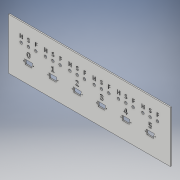
# Autodesk Inventor part: front
Saved by Autodesk Inventor 2017 (Build 210142000, 142)
## iProperties
Created: 2016-09-19
Part Number: front
Material: Generic
Document SubType Name: Modeling
Designer: Darien Morrow
Density: 1 g/cm^3
Appearance: Default
Author: Darien Morrow
Autodesk Inventor part; units mm, degrees
(part 1 of 2)
ref_plane "YZ Plane" through (0, 0, 0) normal (1, 0, 0) x (0, 1, 0)
ref_plane "XZ Plane" through (0, 0, 0) normal (0, 1, 0) x (-1, 0, 0)
ref_plane "XY Plane" through (0, 0, 0) normal (0, 0, 1) x (1, 0, 0)
sketch "Sketch1" plane through (0, 0, 0) normal (0, 0, 1) x (1, 0, 0)
  line L0 (-211.1375, -66.675) -> (211.1375, -66.675)
  line L1 (211.1375, -66.675) -> (211.1375, 66.675)
  line L2 (211.1375, 66.675) -> (-211.1375, 66.675)
  line L3 (-211.1375, 66.675) -> (-211.1375, -66.675)
  line L4 (-211.1375, -66.675) -> (211.1375, 66.675) construction
  line L5 (211.1375, -66.675) -> (-211.1375, 66.675) construction
  point P0 (0, 0)
  dimension "d0" = 133.35
  dimension "d1" = 422.275
  constraints: 12 end point, 2 midpoint, 2 parallel, 1 horizontal, 1 perpendicular
  measures "d0" distance between parallel lines of L0 L2
  measures "d1" distance between parallel lines of L1 L3
extrude "Extrusion1" add sketch "Sketch1" along normal blind 3.175
sketch "Sketch2" plane through (0, 0, 3.175) normal (0, 0, 1) x (1, 0, 0)
  line L0 (211.1375, -66.675) -> (211.1375, 66.675) projected
  line L1 (-211.1375, 19.05) -> (211.1375, 19.05)
  line L2 (211.1375, 19.05) -> (211.1375, -19.05)
  line L3 (211.1375, -19.05) -> (-211.1375, -19.05)
  line L4 (-211.1375, -19.05) -> (-211.1375, 19.05)
  line L5 (-211.1375, 19.05) -> (211.1375, -19.05) construction
  line L6 (211.1375, 19.05) -> (-211.1375, -19.05) construction
  point P0 (0, 0)
  point P1 (19.05, -19.05)
  point P2 (44.45, -19.05)
  point P3 (82.55, -19.05)
  point P4 (107.95, -19.05)
  point P5 (146.05, -19.05)
  point P6 (171.45, -19.05)
  point P7 (-19.05, -19.05)
  point P8 (-44.45, -19.05)
  point P9 (-82.55, -19.05)
  point P10 (-107.95, -19.05)
  point P11 (-146.05, -19.05)
  point P12 (-171.45, -19.05)
  dimension "d4" = 19.05
  dimension "d6" = 25.4
  dimension "d7" = 38.1
  dimension "d8" = 25.4
  dimension "d9" = 38.1
  dimension "d10" = 25.4
  dimension "d12" = 25.4
  dimension "d13" = 38.1
  dimension "d14" = 25.4
  dimension "d15" = 38.1
  dimension "d16" = 25.4
  constraints: 10 end point, 2 horizontal, 2 midpoint, 1 parallel, 1 perpendicular, 1 point on line, 15 other
  measures "d6" distance of point (44.45, -19.05) point (19.05, -19.05)
  measures "d7" distance of point (82.55, -19.05) point (44.45, -19.05)
  measures "d8" distance of point (107.95, -19.05) point (82.55, -19.05)
  measures "d9" distance of point (146.05, -19.05) point (107.95, -19.05)
  measures "d10" distance of point (171.45, -19.05) point (146.05, -19.05)
  measures "d12" distance of point (-44.45, -19.05) point (-19.05, -19.05)
  measures "d13" distance of point (-82.55, -19.05) point (-44.45, -19.05)
  measures "d14" distance of point (-107.95, -19.05) point (-82.55, -19.05)
  measures "d15" distance of point (-146.05, -19.05) point (-107.95, -19.05)
  measures "d16" distance of point (-171.45, -19.05) point (-146.05, -19.05)
hole "Hole1" at (19.05, -19.05, 3.175) at (44.45, -19.05, 3.175) at (82.55, -19.05, 3.175) at (107.95, -19.05, 3.175) at (146.05, -19.05, 3.175) at (171.45, -19.05, 3.175) at (-19.05, -19.05, 3.175) at (-44.45, -19.05, 3.175) at (-82.55, -19.05, 3.175) at (-107.95, -19.05, 3.175) at (-146.05, -19.05, 3.175) at (-171.45, -19.05, 3.175) direction (0, 0, -1) diameter 2.159 end through all
sketch "Sketch3" plane through (0, 0, 3.175) normal (0, 0, 1) x (1, 0, 0)
  circle A0 centre (-146.05, -19.05) radius 1.0795 projected
  line L0 (-211.1375, -66.675) -> (211.1375, -66.675) projected
  line L1 (-167.4813, -25.0031) -> (-150.0188, -25.0031)
  line L2 (-150.0188, -13.0969) -> (-167.4813, -13.0969)
  line L3 (-167.4813, -25.0031) -> (-150.0188, -13.0969) construction
  line L4 (-150.0188, -25.0031) -> (-167.4813, -13.0969) construction
  line L5 (-150.0188, -25.0031) -> (-148.4313, -13.0969)
  line L6 (-167.4813, -25.0031) -> (-169.0688, -13.0969)
  line L7 (-169.0688, -13.0969) -> (-167.4813, -13.0969)
  line L8 (-150.0188, -13.0969) -> (-148.4313, -13.0969)
  line L9 (-161.2761, -3.996) -> (-100.8121, -3.996)
  line L10 (-86.5188, -13.0969) -> (-103.9813, -13.0969)
  line L11 (-105.5688, -13.0969) -> (-103.9813, -13.0969)
  line L12 (-103.9813, -25.0031) -> (-105.5688, -13.0969)
  line L13 (-103.9813, -25.0031) -> (-86.5188, -25.0031)
  line L14 (-86.5188, -25.0031) -> (-84.9313, -13.0969)
  line L15 (-86.5188, -13.0969) -> (-84.9313, -13.0969)
  line L16 (-23.0188, -13.0969) -> (-40.4813, -13.0969)
  line L17 (-42.0688, -13.0969) -> (-40.4813, -13.0969)
  line L18 (-40.4813, -25.0031) -> (-42.0688, -13.0969)
  line L19 (-40.4813, -25.0031) -> (-23.0188, -25.0031)
  line L20 (-23.0188, -25.0031) -> (-21.4313, -13.0969)
  line L21 (-23.0188, -13.0969) -> (-21.4313, -13.0969)
  line L22 (40.4812, -13.0969) -> (23.0187, -13.0969)
  line L23 (21.4312, -13.0969) -> (23.0187, -13.0969)
  line L24 (23.0187, -25.0031) -> (21.4312, -13.0969)
  line L25 (23.0187, -25.0031) -> (40.4812, -25.0031)
  line L26 (40.4812, -25.0031) -> (42.0687, -13.0969)
  line L27 (40.4812, -13.0969) -> (42.0687, -13.0969)
  line L28 (103.9812, -13.0969) -> (86.5187, -13.0969)
  line L29 (84.9312, -13.0969) -> (86.5187, -13.0969)
  line L30 (86.5187, -25.0031) -> (84.9312, -13.0969)
  line L31 (86.5187, -25.0031) -> (103.9812, -25.0031)
  line L32 (103.9812, -25.0031) -> (105.5687, -13.0969)
  line L33 (103.9812, -13.0969) -> (105.5687, -13.0969)
  line L34 (167.4813, -13.0969) -> (150.0187, -13.0969)
  line L35 (148.4312, -13.0969) -> (150.0187, -13.0969)
  line L36 (150.0187, -25.0031) -> (148.4312, -13.0969)
  line L37 (150.0187, -25.0031) -> (167.4813, -25.0031)
  line L38 (167.4813, -25.0031) -> (169.0687, -13.0969)
  line L39 (167.4813, -13.0969) -> (169.0687, -13.0969)
  point P0 (0, 0)
  point P1 (-158.75, -19.05)
  dimension "d24" = 12.7
  dimension "d25" = 47.625
  dimension "d26" = 17.4625
  dimension "d27" = 11.9062
  dimension "d28" = 1.5875
  dimension "d29" = 1.5875
  dimension "d32" = 63.5
  constraints: 78 end point, 4 horizontal, 2 equal length, 2 midpoint, 60 other
  measures "d24" distance of point (-158.75, -19.05) A0.centre
  measures "d25" distance from line of point (-158.75, -19.05) L0
  measures "d26" distance of L2.end L2.start
  measures "d27" distance between parallel lines of L1 L2
  measures "d28" distance of L5.end L2.start
  measures "d29" distance of L2.end L6.end
  measures "d32" distance of L2.start L10.start
extrude "Extrusion2" cut sketch "Sketch3" against normal blind 25.4 contours L6 L7 L2 L8 L5 L1 | L15 L14 L13 L12 L11 L10 | L21 L20 L19 L18 L17 L16 | L27 L26 L25 L24 L23 L22 | L33 L32 L31 L30 L29 L28 | L39 L38 L37 L36 L35 L34
sketch "Sketch4" plane through (0, 0, 3.175) normal (0, 0, 1) x (1, 0, 0)
  line L0 (211.1375, 66.675) -> (-211.1375, 66.675) projected
  line L1 (177.8, -19.05) -> (-177.8, -19.05)
  line L2 (-177.8, -19.05) -> (-177.8, 19.05)
  line L3 (-177.8, 19.05) -> (177.8, 19.05)
  line L4 (177.8, 19.05) -> (177.8, -19.05)
  line L5 (177.8, -19.05) -> (-177.8, 19.05) construction
  line L6 (-177.8, -19.05) -> (177.8, 19.05) construction
  point P0 (0, 0)
  point P1 (-158.75, 19.05)
  point P2 (-139.7, 19.05)
  point P3 (-114.3, 19.05)
  point P4 (-95.25, 19.05)
  point P5 (-76.2, 19.05)
  point P6 (-50.8, 19.05)
  point P7 (-31.75, 19.05)
  point P8 (-12.7, 19.05)
  point P9 (12.7, 19.05)
  point P10 (31.75, 19.05)
  point P11 (50.8, 19.05)
  point P12 (76.2, 19.05)
  point P13 (95.25, 19.05)
  point P14 (114.3, 19.05)
  point P15 (139.7, 19.05)
  point P16 (158.75, 19.05)
  point P17 (177.8, 19.05)
  dimension "d40" = 38.1
  dimension "d41" = 355.6
  dimension "d42" = 19.05
  dimension "d43" = 19.05
  dimension "d46" = 63.5
  constraints: 12 end point, 2 horizontal, 2 midpoint, 2 parallel, 2 point on line, 1 coincident, 1 perpendicular, 15 other
  measures "d40" distance between parallel lines of L1 L3
  measures "d41" distance between parallel lines of L4 L2
  measures "d42" distance of point (-158.75, 19.05) L2.end
  measures "d43" distance of point (-139.7, 19.05) point (-158.75, 19.05)
  measures "d46" distance of L2.end point (-114.3, 19.05)
hole "Hole2" at (-177.8, 19.05, 3.175) at (-158.75, 19.05, 3.175) at (-139.7, 19.05, 3.175) at (-95.25, 19.05, 3.175) at (-76.2, 19.05, 3.175) at (-31.75, 19.05, 3.175) at (-12.7, 19.05, 3.175) at (31.75, 19.05, 3.175) at (50.8, 19.05, 3.175) at (95.25, 19.05, 3.175) at (114.3, 19.05, 3.175) at (158.75, 19.05, 3.175) at (177.8, 19.05, 3.175) at (-50.8, 19.05, 3.175) at (-114.3, 19.05, 3.175) at (12.7, 19.05, 3.175) at (76.2, 19.05, 3.175) at (139.7, 19.05, 3.175) direction (0, 0, -1) diameter 7 end through all
sketch "Sketch5" plane through (0, 0, 3.175) normal (0, 0, 1) x (1, 0, 0)
  line L0 (-163.6339, 6.5797) -> (-140.462, 6.5797) construction
  line L1 (-140.462, 6.5797) -> (-140.462, -4.8632) construction
  line L2 (-140.462, -4.8632) -> (-163.6339, -4.8632) construction
  line L3 (-163.6339, -4.8632) -> (-163.6339, 6.5797) construction
  line L4 (-100.7374, 6.1393) -> (-89.5805, 6.1393) construction
  line L5 (-89.5805, 6.1393) -> (-89.5805, -9.0226) construction
  line L6 (-89.5805, -9.0226) -> (-100.7374, -9.0226) construction
  line L7 (-100.7374, -9.0226) -> (-100.7374, 6.1393) construction
  circle A0 centre (158.75, 19.05) radius 3.5 projected
  line L8 (-211.1375, 66.675) -> (-211.1375, -66.675) projected
  line L9 (-36.8587, 6.6086) -> (-14.4346, 6.6086) construction
  line L10 (-14.4346, 6.6086) -> (-14.4346, -5.5869) construction
  line L11 (-14.4346, -5.5869) -> (-36.8587, -5.5869) construction
  line L12 (-36.8587, -5.5869) -> (-36.8587, 6.6086) construction
  line L13 (27.033, 6.6307) -> (37.1692, 6.6307) construction
  line L14 (37.1692, 6.6307) -> (37.1692, -6.4628) construction
  line L15 (37.1692, -6.4628) -> (27.033, -6.4628) construction
  line L16 (27.033, -6.4628) -> (27.033, 6.6307) construction
  line L17 (89.8174, 6.414) -> (98.2756, 6.414) construction
  line L18 (98.2756, 6.414) -> (98.2756, 0.1196) construction
  line L19 (98.2756, 0.1196) -> (89.8174, 0.1196) construction
  line L20 (89.8174, 0.1196) -> (89.8174, 6.414) construction
  line L21 (153.7586, 6.5556) -> (163.8948, 6.5556) construction
  line L22 (163.8948, 6.5556) -> (163.8948, -6.3113) construction
  line L23 (163.8948, -6.3113) -> (153.7586, -6.3113) construction
  line L24 (153.7586, -6.3113) -> (153.7586, 6.5556) construction
  spline S0 degree 2 poles (-154.0344, 0.0806) (-154.0344, -1.4338) (-154.5233, -3.8784) (-155.6323, -5.5956) (-157.3972, -6.5138) (-158.6731, -6.5138) knots 0 0 0 1 2 3 4 4 4
  spline S1 degree 2 poles (-158.6731, -6.5138) (-159.973, -6.5138) (-161.6782, -5.6195) (-162.668, -3.95) (-163.0734, -1.5412) (-163.0734, -0.0148) knots 0 0 0 1 2 3 4 4 4
  spline S2 degree 2 poles (-163.0734, -0.0148) (-163.0734, 1.4878) (-162.5726, 3.9443) (-161.4755, 5.6615) (-159.6987, 6.5797) (-158.4346, 6.5797) knots 0 0 0 1 2 3 4 4 4
  spline S3 degree 2 poles (-158.4346, 6.5797) (-157.1348, 6.5797) (-155.4177, 5.6853) (-154.4279, 4.0158) (-154.0344, 1.607) (-154.0344, 0.0806) knots 0 0 0 1 2 3 4 4 4
  spline S4 degree 2 poles (-156.6221, -0.0386) (-156.6221, 0.8557) (-156.7175, 2.239) (-156.9202, 3.2526) (-157.2302, 3.9562) (-157.6595, 4.3736) (-158.2081, 4.5525) (-158.542, 4.5525) knots 0 0 0 1 2 3 4 5 6 6 6
  spline S5 degree 2 poles (-158.542, 4.5525) (-159.1144, 4.5525) (-159.8656, 3.992) (-160.3069, 2.883) (-160.4857, 1.2135) (-160.4857, 0.1164) knots 0 0 0 1 2 3 4 4 4
  spline S6 degree 2 poles (-160.4857, 0.1164) (-160.4857, -1.243) (-160.2711, -3.0079) (-159.806, -4.0573) (-159.0905, -4.4747) (-158.5777, -4.4747) knots 0 0 0 1 2 3 4 4 4
  spline S7 degree 2 poles (-158.5777, -4.4747) (-158.1962, -4.4747) (-157.6118, -4.2243) (-157.1706, -3.7353) (-156.8725, -2.996) (-156.6936, -2.0182) (-156.6221, -0.7899) (-156.6221, -0.0386) knots 0 0 0 1 2 3 4 5 6 6 6
  spline S8 degree 2 poles (-91.5075, -5.6186) (-91.5075, -5.8929) (-91.5672, -6.2745) (-91.6745, -6.5011) (-91.8057, -6.5965) (-91.9011, -6.5965) knots 0 0 0 1 2 3 4 4 4
  line L25 (-91.9011, -6.5965) -> (-98.8771, -6.5965)
  spline S9 degree 2 poles (-98.8771, -6.5965) (-98.9606, -6.5965) (-99.0918, -6.5011) (-99.1991, -6.2745) (-99.2587, -5.8929) (-99.2587, -5.6186) knots 0 0 0 1 2 3 4 4 4
  spline S10 degree 2 poles (-99.2587, -5.6186) (-99.2587, -5.3444) (-99.211, -4.9628) (-99.1037, -4.7243) (-98.9606, -4.6169) (-98.8771, -4.6169) knots 0 0 0 1 2 3 4 4 4
  line L26 (-98.8771, -4.6169) -> (-96.5279, -4.6169)
  line L27 (-96.5279, -4.6169) -> (-96.5279, 3.6231)
  line L28 (-96.5279, 3.6231) -> (-98.5671, 2.5022)
  spline S11 degree 2 poles (-98.5671, 2.5022) (-98.7817, 2.3949) (-99.0679, 2.3472) (-99.2349, 2.5141) (-99.2945, 2.9196) (-99.2945, 3.2892) knots 0 0 0 1 2 3 4 4 4
  spline S12 degree 2 poles (-99.2945, 3.2892) (-99.2945, 3.5277) (-99.2706, 3.8259) (-99.1991, 4.0405) (-99.056, 4.1836) (-98.9367, 4.2552) knots 0 0 0 1 2 3 4 4 4
  line L29 (-98.9367, 4.2552) -> (-96.2298, 6.0081)
  spline S13 degree 2 poles (-96.2298, 6.0081) (-96.1702, 6.0558) (-96.0271, 6.1035) (-95.7886, 6.1274) (-95.407, 6.1393) (-95.1088, 6.1393) knots 0 0 0 1 2 3 4 4 4
  spline S14 degree 2 poles (-95.1088, 6.1393) (-94.7392, 6.1393) (-94.2741, 6.1154) (-94.0475, 6.0439) (-93.9641, 5.9246) (-93.9641, 5.8412) knots 0 0 0 1 2 3 4 4 4
  line L30 (-93.9641, 5.8412) -> (-93.9641, -4.6169)
  line L31 (-93.9641, -4.6169) -> (-91.9011, -4.6169)
  spline S15 degree 2 poles (-91.9011, -4.6169) (-91.8057, -4.6169) (-91.6626, -4.7243) (-91.5552, -4.9628) (-91.5075, -5.3444) (-91.5075, -5.6186) knots 0 0 0 1 2 3 4 4 4
  spline S16 degree 2 poles (-27.5215, -5.209) (-27.5215, -5.4952) (-27.5692, -5.9006) (-27.6646, -6.151) (-27.8196, -6.2584) (-27.9269, -6.2584) knots 0 0 0 1 2 3 4 4 4
  line L32 (-27.9269, -6.2584) -> (-35.1892, -6.2584)
  spline S17 degree 2 poles (-35.1892, -6.2584) (-35.4038, -6.2584) (-35.7139, -6.1749) (-35.9166, -5.9602) (-36.0001, -5.519) (-36.0001, -5.1851) knots 0 0 0 1 2 3 4 4 4
  spline S18 degree 2 poles (-36.0001, -5.1851) (-36.0001, -4.8632) (-35.9404, -4.3981) (-35.7854, -4.0403) (-35.535, -3.6945) (-35.3442, -3.4918) knots 0 0 0 1 2 3 4 4 4
  line L33 (-35.3442, -3.4918) -> (-33.1619, -1.1426)
  spline S19 degree 2 poles (-33.1619, -1.1426) (-32.5061, -0.4629) (-31.7071, 0.6581) (-31.254, 1.5882) (-31.087, 2.3633) (-31.087, 2.7211) knots 0 0 0 1 2 3 4 4 4
  spline S20 degree 2 poles (-31.087, 2.7211) (-31.087, 3.043) (-31.2897, 3.6154) (-31.6952, 4.0447) (-32.2914, 4.2952) (-32.7088, 4.2952) knots 0 0 0 1 2 3 4 4 4
  spline S21 degree 2 poles (-32.7088, 4.2952) (-33.2812, 4.2952) (-34.1756, 4.009) (-34.8433, 3.6393) (-35.2965, 3.3412) (-35.4157, 3.3412) knots 0 0 0 1 2 3 4 4 4
  spline S22 degree 2 poles (-35.4157, 3.3412) (-35.5111, 3.3412) (-35.6304, 3.4604) (-35.7139, 3.7347) (-35.7616, 4.1878) (-35.7616, 4.5217) knots 0 0 0 1 2 3 4 4 4
  spline S23 degree 2 poles (-35.7616, 4.5217) (-35.7616, 4.7483) (-35.7377, 5.0583) (-35.6781, 5.273) (-35.5708, 5.4399) (-35.3323, 5.6784) (-34.6764, 6.0362) (-33.7224, 6.382) (-32.5657, 6.6086) (-31.9456, 6.6086) knots 0 0 0 1 2 3 4 5 6 7 8 8 8
  spline S24 degree 2 poles (-31.9456, 6.6086) (-30.9558, 6.6086) (-29.4891, 6.1077) (-28.5112, 5.2253) (-28.0342, 3.997) (-28.0342, 3.2935) knots 0 0 0 1 2 3 4 4 4
  spline S25 degree 2 poles (-28.0342, 3.2935) (-28.0342, 2.6853) (-28.2727, 1.4928) (-29.0121, 0.1095) (-30.3596, -1.56) (-31.4686, -2.6571) knots 0 0 0 1 2 3 4 4 4
  line L34 (-31.4686, -2.6571) -> (-32.9473, -4.1715)
  line L35 (-32.9473, -4.1715) -> (-27.9627, -4.1715)
  spline S26 degree 2 poles (-27.9627, -4.1715) (-27.8673, -4.1715) (-27.7003, -4.2908) (-27.5811, -4.5293) (-27.5215, -4.9347) (-27.5215, -5.209) knots 0 0 0 1 2 3 4 4 4
  spline S27 degree 2 poles (36.3225, -2.5395) (36.3225, -3.4816) (35.5951, -4.9483) (34.3072, -5.95) (32.5065, -6.4628) (31.4452, -6.4628) knots 0 0 0 1 2 3 4 4 4
  spline S28 degree 2 poles (31.4452, -6.4628) (30.8013, -6.4628) (29.6684, -6.272) (28.7979, -6.0096) (28.2255, -5.7115) (28.0586, -5.5565) (27.9632, -5.3538) (27.8916, -5.0914) (27.8678, -4.6979) (27.8678, -4.4117) knots 0 0 0 1 2 3 4 5 6 7 8 8 8
  spline S29 degree 2 poles (27.8678, -4.4117) (27.8678, -3.9347) (28.0228, -3.577) (28.1778, -3.577) knots 0 0 0 1 2 2 2
  spline S30 degree 2 poles (28.1778, -3.577) (28.2732, -3.577) (28.7621, -3.8393) (29.5015, -4.1494) (30.5032, -4.4117) (31.1352, -4.4117) knots 0 0 0 1 2 3 4 4 4
  spline S31 degree 2 poles (31.1352, -4.4117) (31.6718, -4.4117) (32.4946, -4.1613) (33.067, -3.6962) (33.3532, -3.0404) (33.3532, -2.6468) knots 0 0 0 1 2 3 4 4 4
  spline S32 degree 2 poles (33.3532, -2.6468) (33.3532, -2.2056) (33.0074, -1.502) (32.3396, -1.0012) (31.3141, -0.7269) (30.6105, -0.7269) knots 0 0 0 1 2 3 4 4 4
  line L36 (30.6105, -0.7269) -> (29.5134, -0.7269)
  spline S33 degree 2 poles (29.5134, -0.7269) (29.3942, -0.7269) (29.2153, -0.6554) (29.096, -0.4407) (29.0483, -0.0591) (29.0483, 0.239) knots 0 0 0 1 2 3 4 4 4
  spline S34 degree 2 poles (29.0483, 0.239) (29.0483, 0.5252) (29.096, 0.8829) (29.2034, 1.0737) (29.3703, 1.1572) (29.4896, 1.1572) knots 0 0 0 1 2 3 4 4 4
  line L37 (29.4896, 1.1572) -> (30.5986, 1.1572)
  spline S35 degree 2 poles (30.5986, 1.1572) (31.171, 1.1572) (32.0534, 1.4196) (32.6496, 1.9085) (32.9597, 2.6001) (32.9597, 3.0294) knots 0 0 0 1 2 3 4 4 4
  spline S36 degree 2 poles (32.9597, 3.0294) (32.9597, 3.3514) (32.745, 3.9238) (32.3277, 4.3412) (31.6599, 4.5916) (31.2067, 4.5916) knots 0 0 0 1 2 3 4 4 4
  spline S37 degree 2 poles (31.2067, 4.5916) (30.694, 4.5916) (29.7996, 4.2935) (29.0841, 3.9238) (28.5833, 3.6137) (28.464, 3.6137) knots 0 0 0 1 2 3 4 4 4
  spline S38 degree 2 poles (28.464, 3.6137) (28.3925, 3.6137) (28.2732, 3.6853) (28.1897, 3.8761) (28.154, 4.2458) (28.154, 4.5439) knots 0 0 0 1 2 3 4 4 4
  spline S39 degree 2 poles (28.154, 4.5439) (28.154, 4.7824) (28.1778, 5.1043) (28.2374, 5.319) (28.3209, 5.474) (28.5117, 5.6648) (29.1199, 6.0345) (30.0381, 6.3922) (31.2425, 6.6307) (31.9461, 6.6307) knots 0 0 0 1 2 3 4 5 6 7 8 8 8
  spline S40 degree 2 poles (31.9461, 6.6307) (32.8643, 6.6307) (34.2834, 6.2014) (35.2493, 5.3905) (35.7501, 4.21) (35.7501, 3.4587) knots 0 0 0 1 2 3 4 4 4
  spline S41 degree 2 poles (35.7501, 3.4587) (35.7501, 2.8863) (35.452, 1.8965) (34.8915, 1.1095) (34.0329, 0.561) (33.4844, 0.4298) knots 0 0 0 1 2 3 4 4 4
  line L38 (33.4844, 0.4298) -> (33.4844, 0.394)
  spline S42 degree 2 poles (33.4844, 0.394) (34.1403, 0.3225) (35.2016, -0.2022) (35.929, -0.9773) (36.3225, -1.9671) (36.3225, -2.5395) knots 0 0 0 1 2 3 4 4 4
  spline S43 degree 2 poles (99.5601, -2.6608) (99.5601, -3.1616) (99.3573, -3.6744) (99.1785, -3.6744) knots 0 0 0 1 2 2 2
  line L39 (99.1785, -3.6744) -> (98.0575, -3.6744)
  line L40 (98.0575, -3.6744) -> (98.0575, -5.9521)
  spline S44 degree 2 poles (98.0575, -5.9521) (98.0575, -6.0475) (97.9383, -6.2025) (97.6521, -6.2979) (97.1751, -6.3456) (96.8054, -6.3456) knots 0 0 0 1 2 3 4 4 4
  spline S45 degree 2 poles (96.8054, -6.3456) (96.4596, -6.3456) (95.9826, -6.2979) (95.6964, -6.2025) (95.5891, -6.0475) (95.5891, -5.9521) knots 0 0 0 1 2 3 4 4 4
  line L41 (95.5891, -5.9521) -> (95.5891, -3.6744)
  line L42 (95.5891, -3.6744) -> (90.7476, -3.6744)
  spline S46 degree 2 poles (90.7476, -3.6744) (90.6045, -3.6744) (90.3898, -3.6029) (90.2467, -3.3644) (90.1752, -2.8993) (90.1752, -2.5177) knots 0 0 0 1 2 3 4 4 4
  spline S47 degree 2 poles (90.1752, -2.5177) (90.1752, -2.2076) (90.199, -1.7545) (90.2706, -1.3729) (90.4018, -1.0509) (90.4972, -0.8601) knots 0 0 0 1 2 3 4 4 4
  line L43 (90.4972, -0.8601) -> (94.4324, 6.0682)
  spline S48 degree 2 poles (94.4324, 6.0682) (94.4801, 6.1636) (94.7186, 6.2829) (95.1359, 6.3783) (95.7799, 6.414) (96.245, 6.414) knots 0 0 0 1 2 3 4 4 4
  spline S49 degree 2 poles (96.245, 6.414) (96.7458, 6.414) (97.4374, 6.3663) (97.8667, 6.259) (98.0575, 6.104) (98.0575, 5.9967) knots 0 0 0 1 2 3 4 4 4
  line L44 (98.0575, 5.9967) -> (98.0575, -1.6233)
  line L45 (98.0575, -1.6233) -> (99.1785, -1.6233)
  spline S50 degree 2 poles (99.1785, -1.6233) (99.3335, -1.6233) (99.5601, -2.1003) (99.5601, -2.6608) knots 0 0 0 1 2 2 2
  line L46 (95.5891, 4.196) -> (95.5652, 4.196)
  line L47 (95.5652, 4.196) -> (92.2263, -1.6233)
  line L48 (92.2263, -1.6233) -> (95.5891, -1.6233)
  line L49 (95.5891, -1.6233) -> (95.5891, 4.196)
  spline S51 degree 2 poles (162.9885, -1.9826) (162.9885, -3.0081) (162.273, -4.618) (160.9732, -5.727) (159.1487, -6.3113) (158.0277, -6.3113) knots 0 0 0 1 2 3 4 4 4
  spline S52 degree 2 poles (158.0277, -6.3113) (157.4434, -6.3113) (156.394, -6.1682) (155.5473, -5.9417) (155.0107, -5.7151) (154.8438, -5.572) (154.7722, -5.3931) (154.7245, -5.1427) (154.7007, -4.773) (154.7007, -4.5226) knots 0 0 0 1 2 3 4 5 6 7 8 8 8
  spline S53 degree 2 poles (154.7007, -4.5226) (154.7007, -4.2483) (154.7365, -3.8667) (154.8319, -3.6282) (154.9392, -3.5328) (155.0227, -3.5328) knots 0 0 0 1 2 3 4 4 4
  spline S54 degree 2 poles (155.0227, -3.5328) (155.1181, -3.5328) (155.5235, -3.7594) (156.1794, -4.0337) (157.1095, -4.2603) (157.7654, -4.2603) knots 0 0 0 1 2 3 4 4 4
  spline S55 degree 2 poles (157.7654, -4.2603) (158.3378, -4.2603) (159.256, -4.0218) (159.9119, -3.509) (160.2577, -2.722) (160.2577, -2.1853) knots 0 0 0 1 2 3 4 4 4
  spline S56 degree 2 poles (160.2577, -2.1853) (160.2577, -1.7083) (159.9596, -0.9809) (159.3395, -0.4681) (158.3497, -0.2177) (157.6342, -0.2177) knots 0 0 0 1 2 3 4 4 4
  spline S57 degree 2 poles (157.6342, -0.2177) (157.0618, -0.2177) (156.1436, -0.337) (155.7262, -0.337) knots 0 0 0 1 2 2 2
  spline S58 degree 2 poles (155.7262, -0.337) (155.44, -0.337) (155.2015, -0.0508) (155.2015, 0.3308) knots 0 0 0 1 2 2 2
  line L50 (155.2015, 0.3308) -> (155.2015, 5.8282)
  spline S59 degree 2 poles (155.2015, 5.8282) (155.2015, 6.2098) (155.4996, 6.5556) (155.8335, 6.5556) knots 0 0 0 1 2 2 2
  line L51 (155.8335, 6.5556) -> (161.8198, 6.5556)
  spline S60 degree 2 poles (161.8198, 6.5556) (161.9152, 6.5556) (162.0703, 6.4364) (162.1776, 6.1859) (162.2253, 5.7686) (162.2253, 5.4704) knots 0 0 0 1 2 3 4 4 4
  spline S61 degree 2 poles (162.2253, 5.4704) (162.2253, 4.8861) (162.0226, 4.3614) (161.8198, 4.3614) knots 0 0 0 1 2 2 2
  line L52 (161.8198, 4.3614) -> (157.3361, 4.3614)
  line L53 (157.3361, 4.3614) -> (157.3361, 1.6426)
  spline S62 degree 2 poles (157.3361, 1.6426) (157.6819, 1.6783) (158.3497, 1.7022) (158.7194, 1.7022) knots 0 0 0 1 2 2 2
  spline S63 degree 2 poles (158.7194, 1.7022) (159.7449, 1.7022) (161.3428, 1.2252) (162.428, 0.295) (162.9885, -1.0763) (162.9885, -1.9826) knots 0 0 0 1 2 3 4 4 4
  point P0 (0, 0)
  constraints: 12 other
emboss "Emboss1" sketch "Sketch5" operation cut depth 1.27 direction (0, 0, -1) contours S0 S1 S2 S3 | S8 L25 S9 S10 L26 L27 L28 S11 S12 L29 S13 S14 L30 L31 S15 | S16 L32 S17 S18 L33 S19 S20 S21 S22 S23 S24 S25 L34 L35 S26 | S27 S28 S29 S30 S31 S32 L36 S33 S34 L37 S35 S36 S37 S38 S39 S40 S41 L38 S42 | S43 L39 L40 S44 S45 L41 L42 S46 S47 L43 S48 S49 L44 L45 S50 | S51 S52 S53 S54 S55 S56 S57 S58 L50 S59 L51 S60 S61 L52 L53 S62 S63
sketch "Sketch6" plane through (0, 0, 3.175) normal (0, 0, 1) x (1, 0, 0)
  line L0 (-182.5364, 38.2905) -> (-176.4863, 38.2905) construction
  line L1 (-176.4863, 38.2905) -> (-176.4863, 32.7976) construction
  line L2 (-176.4863, 32.7976) -> (-182.5364, 32.7976) construction
  line L3 (-182.5364, 32.7976) -> (-182.5364, 38.2905) construction
  line L4 (-162.3961, 38.6089) -> (-155.3038, 38.6089) construction
  line L5 (-155.3038, 38.6089) -> (-155.3038, 28.7887) construction
  line L6 (-155.3038, 28.7887) -> (-162.3961, 28.7887) construction
  line L7 (-162.3961, 28.7887) -> (-162.3961, 38.6089) construction
  line L8 (-142.813, 38.2108) -> (-135.9264, 38.2108) construction
  line L9 (-135.9264, 38.2108) -> (-135.9264, 28.6858) construction
  line L10 (-135.9264, 28.6858) -> (-142.813, 28.6858) construction
  line L11 (-142.813, 28.6858) -> (-142.813, 38.2108) construction
  line L12 (-118.6971, 38.2858) -> (-112.647, 38.2858) construction
  line L13 (-112.647, 38.2858) -> (-112.647, 32.793) construction
  line L14 (-112.647, 32.793) -> (-118.6971, 32.793) construction
  line L15 (-118.6971, 32.793) -> (-118.6971, 38.2858) construction
  line L16 (-98.5568, 38.6043) -> (-91.4644, 38.6043) construction
  line L17 (-91.4644, 38.6043) -> (-91.4644, 28.7841) construction
  line L18 (-91.4644, 28.7841) -> (-98.5568, 28.7841) construction
  line L19 (-98.5568, 28.7841) -> (-98.5568, 38.6043) construction
  line L20 (-78.9737, 38.2062) -> (-72.0871, 38.2062) construction
  line L21 (-72.0871, 38.2062) -> (-72.0871, 28.6812) construction
  line L22 (-72.0871, 28.6812) -> (-78.9737, 28.6812) construction
  line L23 (-78.9737, 28.6812) -> (-78.9737, 38.2062) construction
  line L24 (211.1375, -66.675) -> (211.1375, 66.675) projected
  circle A0 centre (12.7, 19.05) radius 3.5 projected
  line L25 (-15.5126, 28.7583) -> (-15.5126, 38.2833) construction
  line L26 (-15.5126, 38.2833) -> (-8.626, 38.2833) construction
  line L27 (-8.626, 38.2833) -> (-8.626, 28.7583) construction
  line L28 (-8.626, 28.7583) -> (-15.5126, 28.7583) construction
  line L29 (-35.0957, 28.8612) -> (-35.0957, 38.6813) construction
  line L30 (-35.0957, 38.6813) -> (-28.0033, 38.6813) construction
  line L31 (-28.0033, 38.6813) -> (-28.0033, 28.8612) construction
  line L32 (-28.0033, 28.8612) -> (-35.0957, 28.8612) construction
  line L33 (-55.236, 32.8701) -> (-55.236, 38.3629) construction
  line L34 (-55.236, 38.3629) -> (-49.1859, 38.3629) construction
  line L35 (-49.1859, 38.3629) -> (-49.1859, 32.8701) construction
  line L36 (-49.1859, 32.8701) -> (-55.236, 32.8701) construction
  line L37 (8.0094, 32.7314) -> (8.0094, 38.2242) construction
  line L38 (8.0094, 38.2242) -> (14.0594, 38.2242) construction
  line L39 (14.0594, 38.2242) -> (14.0594, 32.7314) construction
  line L40 (14.0594, 32.7314) -> (8.0094, 32.7314) construction
  line L41 (28.1497, 28.7225) -> (28.1497, 38.5426) construction
  line L42 (28.1497, 38.5426) -> (35.242, 38.5426) construction
  line L43 (35.242, 38.5426) -> (35.242, 28.7225) construction
  line L44 (35.242, 28.7225) -> (28.1497, 28.7225) construction
  line L45 (47.7327, 28.6196) -> (47.7327, 38.1446) construction
  line L46 (47.7327, 38.1446) -> (54.6193, 38.1446) construction
  line L47 (54.6193, 38.1446) -> (54.6193, 28.6196) construction
  line L48 (54.6193, 28.6196) -> (47.7327, 28.6196) construction
  line L49 (111.3017, 28.6967) -> (111.3017, 38.2217) construction
  line L50 (111.3017, 38.2217) -> (118.1883, 38.2217) construction
  line L51 (118.1883, 38.2217) -> (118.1883, 28.6967) construction
  line L52 (118.1883, 28.6967) -> (111.3017, 28.6967) construction
  line L53 (91.7186, 28.7996) -> (91.7186, 38.6197) construction
  line L54 (91.7186, 38.6197) -> (98.811, 38.6197) construction
  line L55 (98.811, 38.6197) -> (98.811, 28.7996) construction
  line L56 (98.811, 28.7996) -> (91.7186, 28.7996) construction
  line L57 (71.5783, 32.8085) -> (71.5783, 38.3013) construction
  line L58 (71.5783, 38.3013) -> (77.6284, 38.3013) construction
  line L59 (77.6284, 38.3013) -> (77.6284, 32.8085) construction
  line L60 (77.6284, 32.8085) -> (71.5783, 32.8085) construction
  line L61 (135.0934, 32.7237) -> (135.0934, 38.2165) construction
  line L62 (135.0934, 38.2165) -> (141.1434, 38.2165) construction
  line L63 (141.1434, 38.2165) -> (141.1434, 32.7237) construction
  line L64 (141.1434, 32.7237) -> (135.0934, 32.7237) construction
  line L65 (155.2337, 28.7148) -> (155.2337, 38.5349) construction
  line L66 (155.2337, 38.5349) -> (162.326, 38.5349) construction
  line L67 (162.326, 38.5349) -> (162.326, 28.7148) construction
  line L68 (162.326, 28.7148) -> (155.2337, 28.7148) construction
  line L69 (174.8167, 28.6119) -> (174.8167, 38.1369) construction
  line L70 (174.8167, 38.1369) -> (181.7033, 38.1369) construction
  line L71 (181.7033, 38.1369) -> (181.7033, 28.6119) construction
  line L72 (181.7033, 28.6119) -> (174.8167, 28.6119) construction
  spline S0 degree 2 poles (-174.0936, 29.0248) (-174.0936, 28.9533) (-174.192, 28.837) (-174.4066, 28.7655) (-174.7733, 28.7207) (-175.0505, 28.7207) knots 0 0 0 1 2 3 4 4 4
  spline S1 degree 2 poles (-175.0505, 28.7207) (-175.3367, 28.7207) (-175.7124, 28.7655) (-175.9181, 28.837) (-176.0165, 28.9533) (-176.0165, 29.0248) knots 0 0 0 1 2 3 4 4 4
  line L73 (-176.0165, 29.0248) -> (-176.0165, 32.8616)
  line L74 (-176.0165, 32.8616) -> (-179.576, 32.8616)
  line L75 (-179.576, 32.8616) -> (-179.576, 29.0248)
  spline S2 degree 2 poles (-179.576, 29.0248) (-179.576, 28.9533) (-179.6655, 28.837) (-179.8801, 28.7655) (-180.2468, 28.7207) (-180.533, 28.7207) knots 0 0 0 1 2 3 4 4 4
  spline S3 degree 2 poles (-180.533, 28.7207) (-180.8103, 28.7207) (-181.1859, 28.7655) (-181.4005, 28.837) (-181.4989, 28.9533) (-181.4989, 29.0248) knots 0 0 0 1 2 3 4 4 4
  line L76 (-181.4989, 29.0248) -> (-181.4989, 37.9864)
  spline S4 degree 2 poles (-181.4989, 37.9864) (-181.4989, 38.0579) (-181.4005, 38.1742) (-181.1859, 38.2457) (-180.8103, 38.2905) (-180.533, 38.2905) knots 0 0 0 1 2 3 4 4 4
  spline S5 degree 2 poles (-180.533, 38.2905) (-180.2468, 38.2905) (-179.8801, 38.2457) (-179.6655, 38.1742) (-179.576, 38.0579) (-179.576, 37.9864) knots 0 0 0 1 2 3 4 4 4
  line L77 (-179.576, 37.9864) -> (-179.576, 34.5073)
  line L78 (-179.576, 34.5073) -> (-176.0165, 34.5073)
  line L79 (-176.0165, 34.5073) -> (-176.0165, 37.9864)
  spline S6 degree 2 poles (-176.0165, 37.9864) (-176.0165, 38.0579) (-175.9181, 38.1742) (-175.7124, 38.2457) (-175.3367, 38.2905) (-175.0505, 38.2905) knots 0 0 0 1 2 3 4 4 4
  spline S7 degree 2 poles (-175.0505, 38.2905) (-174.7733, 38.2905) (-174.4066, 38.2457) (-174.192, 38.1742) (-174.0936, 38.0579) (-174.0936, 37.9864) knots 0 0 0 1 2 3 4 4 4
  line L80 (-174.0936, 37.9864) -> (-174.0936, 29.0248)
  spline S8 degree 2 poles (-91.9027, 31.7981) (-91.9027, 31.0469) (-92.4572, 29.92) (-93.4142, 29.1687) (-94.6842, 28.7841) (-95.4086, 28.7841) knots 0 0 0 1 2 3 4 4 4
  spline S9 degree 2 poles (-95.4086, 28.7841) (-95.9005, 28.7841) (-96.7412, 28.9451) (-97.3851, 29.1776) (-97.8234, 29.4281) (-98.0112, 29.6159) (-98.0917, 29.9736) (-98.0917, 30.3135) knots 0 0 0 1 2 3 4 5 6 6 6
  spline S10 degree 2 poles (-98.0917, 30.3135) (-98.0917, 30.5371) (-98.0649, 30.8501) (-97.9933, 31.0379) (-97.886, 31.1184) (-97.8144, 31.1184) knots 0 0 0 1 2 3 4 4 4
  spline S11 degree 2 poles (-97.8144, 31.1184) (-97.7071, 31.1184) (-97.3404, 30.8769) (-96.7501, 30.5818) (-95.9363, 30.3403) (-95.4086, 30.3403) knots 0 0 0 1 2 3 4 4 4
  spline S12 degree 2 poles (-95.4086, 30.3403) (-95.0508, 30.3403) (-94.4963, 30.5102) (-94.1118, 30.8143) (-93.9061, 31.2705) (-93.9061, 31.5477) knots 0 0 0 1 2 3 4 4 4
  spline S13 degree 2 poles (-93.9061, 31.5477) (-93.9061, 31.8697) (-94.2549, 32.3347) (-94.8183, 32.6925) (-95.5338, 33.0055) (-96.303, 33.3543) (-97.0184, 33.8015) (-97.5819, 34.4276) (-97.9307, 35.2772) (-97.9307, 35.8675) knots 0 0 0 1 2 3 4 5 6 7 8 8 8
  spline S14 degree 2 poles (-97.9307, 35.8675) (-97.9307, 36.5562) (-97.4209, 37.5847) (-96.5713, 38.2644) (-95.3996, 38.6043) (-94.7468, 38.6043) knots 0 0 0 1 2 3 4 4 4
  spline S15 degree 2 poles (-94.7468, 38.6043) (-94.4158, 38.6043) (-93.7361, 38.5059) (-93.1548, 38.327) (-92.6987, 38.1034) (-92.5466, 37.9603) (-92.5019, 37.8619) (-92.4661, 37.692) (-92.4482, 37.4326) (-92.4482, 37.2448) knots 0 0 0 1 2 3 4 5 6 7 8 8 8
  spline S16 degree 2 poles (-92.4482, 37.2448) (-92.4482, 37.0302) (-92.4661, 36.735) (-92.5198, 36.5472) (-92.6182, 36.4578) (-92.6987, 36.4578) knots 0 0 0 1 2 3 4 4 4
  spline S17 degree 2 poles (-92.6987, 36.4578) (-92.7792, 36.4578) (-93.128, 36.6635) (-93.6467, 36.905) (-94.3175, 37.1017) (-94.7199, 37.1017) knots 0 0 0 1 2 3 4 4 4
  spline S18 degree 2 poles (-94.7199, 37.1017) (-95.033, 37.1017) (-95.507, 36.9497) (-95.82, 36.6724) (-95.972, 36.2968) (-95.972, 36.0821) knots 0 0 0 1 2 3 4 4 4
  spline S19 degree 2 poles (-95.972, 36.0821) (-95.972, 35.7691) (-95.6322, 35.304) (-95.0508, 34.9463) (-94.3175, 34.6333) (-93.5572, 34.2845) (-92.8239, 33.8373) (-92.2515, 33.2112) (-91.9027, 32.3705) (-91.9027, 31.7981) knots 0 0 0 1 2 3 4 5 6 7 8 8 8
  spline S20 degree 2 poles (-110.2542, 29.0202) (-110.2542, 28.9486) (-110.3526, 28.8324) (-110.5673, 28.7608) (-110.934, 28.7161) (-111.2112, 28.7161) knots 0 0 0 1 2 3 4 4 4
  spline S21 degree 2 poles (-111.2112, 28.7161) (-111.4974, 28.7161) (-111.873, 28.7608) (-112.0787, 28.8324) (-112.1771, 28.9486) (-112.1771, 29.0202) knots 0 0 0 1 2 3 4 4 4
  line L81 (-112.1771, 29.0202) -> (-112.1771, 32.857)
  line L82 (-112.1771, 32.857) -> (-115.7367, 32.857)
  line L83 (-115.7367, 32.857) -> (-115.7367, 29.0202)
  spline S22 degree 2 poles (-115.7367, 29.0202) (-115.7367, 28.9486) (-115.8261, 28.8324) (-116.0408, 28.7608) (-116.4075, 28.7161) (-116.6937, 28.7161) knots 0 0 0 1 2 3 4 4 4
  spline S23 degree 2 poles (-116.6937, 28.7161) (-116.9709, 28.7161) (-117.3466, 28.7608) (-117.5612, 28.8324) (-117.6596, 28.9486) (-117.6596, 29.0202) knots 0 0 0 1 2 3 4 4 4
  line L84 (-117.6596, 29.0202) -> (-117.6596, 37.9817)
  spline S24 degree 2 poles (-117.6596, 37.9817) (-117.6596, 38.0533) (-117.5612, 38.1696) (-117.3466, 38.2411) (-116.9709, 38.2858) (-116.6937, 38.2858) knots 0 0 0 1 2 3 4 4 4
  spline S25 degree 2 poles (-116.6937, 38.2858) (-116.4075, 38.2858) (-116.0408, 38.2411) (-115.8261, 38.1696) (-115.7367, 38.0533) (-115.7367, 37.9817) knots 0 0 0 1 2 3 4 4 4
  line L85 (-115.7367, 37.9817) -> (-115.7367, 34.5027)
  line L86 (-115.7367, 34.5027) -> (-112.1771, 34.5027)
  line L87 (-112.1771, 34.5027) -> (-112.1771, 37.9817)
  spline S26 degree 2 poles (-112.1771, 37.9817) (-112.1771, 38.0533) (-112.0787, 38.1696) (-111.873, 38.2411) (-111.4974, 38.2858) (-111.2112, 38.2858) knots 0 0 0 1 2 3 4 4 4
  spline S27 degree 2 poles (-111.2112, 38.2858) (-110.934, 38.2858) (-110.5673, 38.2411) (-110.3526, 38.1696) (-110.2542, 38.0533) (-110.2542, 37.9817) knots 0 0 0 1 2 3 4 4 4
  line L88 (-110.2542, 37.9817) -> (-110.2542, 29.0202)
  spline S28 degree 2 poles (-136.4541, 37.4238) (-136.4541, 37.2002) (-136.4899, 36.8961) (-136.5704, 36.7262) (-136.6777, 36.6368) (-136.7403, 36.6368) knots 0 0 0 1 2 3 4 4 4
  line L89 (-136.7403, 36.6368) -> (-139.8437, 36.6368)
  line L90 (-139.8437, 36.6368) -> (-139.8437, 34.0878)
  line L91 (-139.8437, 34.0878) -> (-136.9281, 34.0878)
  spline S29 degree 2 poles (-136.9281, 34.0878) (-136.8655, 34.0878) (-136.7582, 34.0163) (-136.6777, 33.8374) (-136.6419, 33.5423) (-136.6419, 33.3276) knots 0 0 0 1 2 3 4 4 4
  spline S30 degree 2 poles (-136.6419, 33.3276) (-136.6419, 33.104) (-136.6777, 32.8089) (-136.7582, 32.6211) (-136.8655, 32.5406) (-136.9281, 32.5406) knots 0 0 0 1 2 3 4 4 4
  line L92 (-136.9281, 32.5406) -> (-139.8437, 32.5406)
  line L93 (-139.8437, 32.5406) -> (-139.8437, 29.0078)
  spline S31 degree 2 poles (-139.8437, 29.0078) (-139.8437, 28.9273) (-139.9332, 28.8111) (-140.1568, 28.7306) (-140.5235, 28.6858) (-140.8097, 28.6858) knots 0 0 0 1 2 3 4 4 4
  spline S32 degree 2 poles (-140.8097, 28.6858) (-141.0869, 28.6858) (-141.4625, 28.7306) (-141.6772, 28.8111) (-141.7756, 28.9273) (-141.7756, 29.0078) knots 0 0 0 1 2 3 4 4 4
  line L94 (-141.7756, 29.0078) -> (-141.7756, 37.6027)
  spline S33 degree 2 poles (-141.7756, 37.6027) (-141.7756, 37.9246) (-141.4447, 38.2108) (-141.2032, 38.2108) knots 0 0 0 1 2 2 2
  line L95 (-141.2032, 38.2108) -> (-136.7403, 38.2108)
  spline S34 degree 2 poles (-136.7403, 38.2108) (-136.6777, 38.2108) (-136.5704, 38.1304) (-136.4899, 37.9515) (-136.4541, 37.6385) (-136.4541, 37.4238) knots 0 0 0 1 2 3 4 4 4
  spline S35 degree 2 poles (-155.742, 31.8027) (-155.742, 31.0515) (-156.2965, 29.9246) (-157.2535, 29.1733) (-158.5235, 28.7887) (-159.2479, 28.7887) knots 0 0 0 1 2 3 4 4 4
  spline S36 degree 2 poles (-159.2479, 28.7887) (-159.7398, 28.7887) (-160.5805, 28.9497) (-161.2245, 29.1823) (-161.6627, 29.4327) (-161.8505, 29.6205) (-161.931, 29.9782) (-161.931, 30.3181) knots 0 0 0 1 2 3 4 5 6 6 6
  spline S37 degree 2 poles (-161.931, 30.3181) (-161.931, 30.5417) (-161.9042, 30.8547) (-161.8326, 31.0425) (-161.7253, 31.123) (-161.6538, 31.123) knots 0 0 0 1 2 3 4 4 4
  spline S38 degree 2 poles (-161.6538, 31.123) (-161.5464, 31.123) (-161.1798, 30.8816) (-160.5895, 30.5864) (-159.7756, 30.3449) (-159.2479, 30.3449) knots 0 0 0 1 2 3 4 4 4
  spline S39 degree 2 poles (-159.2479, 30.3449) (-158.8902, 30.3449) (-158.3357, 30.5149) (-157.9511, 30.8189) (-157.7454, 31.2751) (-157.7454, 31.5523) knots 0 0 0 1 2 3 4 4 4
  spline S40 degree 2 poles (-157.7454, 31.5523) (-157.7454, 31.8743) (-158.0942, 32.3394) (-158.6576, 32.6971) (-159.3731, 33.0101) (-160.1423, 33.3589) (-160.8578, 33.8061) (-161.4212, 34.4322) (-161.77, 35.2818) (-161.77, 35.8721) knots 0 0 0 1 2 3 4 5 6 7 8 8 8
  spline S41 degree 2 poles (-161.77, 35.8721) (-161.77, 36.5608) (-161.2602, 37.5893) (-160.4106, 38.269) (-159.239, 38.6089) (-158.5861, 38.6089) knots 0 0 0 1 2 3 4 4 4
  spline S42 degree 2 poles (-158.5861, 38.6089) (-158.2552, 38.6089) (-157.5755, 38.5105) (-156.9941, 38.3316) (-156.538, 38.108) (-156.3859, 37.9649) (-156.3412, 37.8666) (-156.3055, 37.6966) (-156.2876, 37.4373) (-156.2876, 37.2494) knots 0 0 0 1 2 3 4 5 6 7 8 8 8
  spline S43 degree 2 poles (-156.2876, 37.2494) (-156.2876, 37.0348) (-156.3055, 36.7396) (-156.3591, 36.5518) (-156.4575, 36.4624) (-156.538, 36.4624) knots 0 0 0 1 2 3 4 4 4
  spline S44 degree 2 poles (-156.538, 36.4624) (-156.6185, 36.4624) (-156.9673, 36.6681) (-157.486, 36.9096) (-158.1568, 37.1063) (-158.5593, 37.1063) knots 0 0 0 1 2 3 4 4 4
  spline S45 degree 2 poles (-158.5593, 37.1063) (-158.8723, 37.1063) (-159.3463, 36.9543) (-159.6593, 36.677) (-159.8114, 36.3014) (-159.8114, 36.0868) knots 0 0 0 1 2 3 4 4 4
  spline S46 degree 2 poles (-159.8114, 36.0868) (-159.8114, 35.7737) (-159.4715, 35.3087) (-158.8902, 34.9509) (-158.1568, 34.6379) (-157.3966, 34.2891) (-156.6632, 33.8419) (-156.0908, 33.2158) (-155.742, 32.3751) (-155.742, 31.8027) knots 0 0 0 1 2 3 4 5 6 7 8 8 8
  spline S47 degree 2 poles (-72.6148, 37.4192) (-72.6148, 37.1956) (-72.6505, 36.8915) (-72.731, 36.7216) (-72.8383, 36.6321) (-72.901, 36.6321) knots 0 0 0 1 2 3 4 4 4
  line L96 (-72.901, 36.6321) -> (-76.0044, 36.6321)
  line L97 (-76.0044, 36.6321) -> (-76.0044, 34.0832)
  line L98 (-76.0044, 34.0832) -> (-73.0888, 34.0832)
  spline S48 degree 2 poles (-73.0888, 34.0832) (-73.0262, 34.0832) (-72.9188, 34.0116) (-72.8383, 33.8328) (-72.8026, 33.5376) (-72.8026, 33.323) knots 0 0 0 1 2 3 4 4 4
  spline S49 degree 2 poles (-72.8026, 33.323) (-72.8026, 33.0994) (-72.8383, 32.8043) (-72.9188, 32.6164) (-73.0262, 32.5359) (-73.0888, 32.5359) knots 0 0 0 1 2 3 4 4 4
  line L99 (-73.0888, 32.5359) -> (-76.0044, 32.5359)
  line L100 (-76.0044, 32.5359) -> (-76.0044, 29.0032)
  spline S50 degree 2 poles (-76.0044, 29.0032) (-76.0044, 28.9227) (-76.0938, 28.8064) (-76.3174, 28.7259) (-76.6841, 28.6812) (-76.9703, 28.6812) knots 0 0 0 1 2 3 4 4 4
  spline S51 degree 2 poles (-76.9703, 28.6812) (-77.2476, 28.6812) (-77.6232, 28.7259) (-77.8379, 28.8064) (-77.9362, 28.9227) (-77.9362, 29.0032) knots 0 0 0 1 2 3 4 4 4
  line L101 (-77.9362, 29.0032) -> (-77.9362, 37.5981)
  spline S52 degree 2 poles (-77.9362, 37.5981) (-77.9362, 37.92) (-77.6053, 38.2062) (-77.3638, 38.2062) knots 0 0 0 1 2 2 2
  line L102 (-77.3638, 38.2062) -> (-72.901, 38.2062)
  spline S53 degree 2 poles (-72.901, 38.2062) (-72.8383, 38.2062) (-72.731, 38.1257) (-72.6505, 37.9469) (-72.6148, 37.6338) (-72.6148, 37.4192) knots 0 0 0 1 2 3 4 4 4
  spline S54 degree 2 poles (-46.7931, 29.0973) (-46.7931, 29.0257) (-46.8915, 28.9095) (-47.1062, 28.8379) (-47.4729, 28.7932) (-47.7501, 28.7932) knots 0 0 0 1 2 3 4 4 4
  spline S55 degree 2 poles (-47.7501, 28.7932) (-48.0363, 28.7932) (-48.4119, 28.8379) (-48.6177, 28.9095) (-48.716, 29.0257) (-48.716, 29.0973) knots 0 0 0 1 2 3 4 4 4
  line L103 (-48.716, 29.0973) -> (-48.716, 32.9341)
  line L104 (-48.716, 32.9341) -> (-52.2756, 32.9341)
  line L105 (-52.2756, 32.9341) -> (-52.2756, 29.0973)
  spline S56 degree 2 poles (-52.2756, 29.0973) (-52.2756, 29.0257) (-52.365, 28.9095) (-52.5797, 28.8379) (-52.9464, 28.7932) (-53.2326, 28.7932) knots 0 0 0 1 2 3 4 4 4
  spline S57 degree 2 poles (-53.2326, 28.7932) (-53.5098, 28.7932) (-53.8855, 28.8379) (-54.1001, 28.9095) (-54.1985, 29.0257) (-54.1985, 29.0973) knots 0 0 0 1 2 3 4 4 4
  line L106 (-54.1985, 29.0973) -> (-54.1985, 38.0588)
  spline S58 degree 2 poles (-54.1985, 38.0588) (-54.1985, 38.1304) (-54.1001, 38.2466) (-53.8855, 38.3182) (-53.5098, 38.3629) (-53.2326, 38.3629) knots 0 0 0 1 2 3 4 4 4
  spline S59 degree 2 poles (-53.2326, 38.3629) (-52.9464, 38.3629) (-52.5797, 38.3182) (-52.365, 38.2466) (-52.2756, 38.1304) (-52.2756, 38.0588) knots 0 0 0 1 2 3 4 4 4
  line L107 (-52.2756, 38.0588) -> (-52.2756, 34.5797)
  line L108 (-52.2756, 34.5797) -> (-48.716, 34.5797)
  line L109 (-48.716, 34.5797) -> (-48.716, 38.0588)
  spline S60 degree 2 poles (-48.716, 38.0588) (-48.716, 38.1304) (-48.6177, 38.2466) (-48.4119, 38.3182) (-48.0363, 38.3629) (-47.7501, 38.3629) knots 0 0 0 1 2 3 4 4 4
  spline S61 degree 2 poles (-47.7501, 38.3629) (-47.4729, 38.3629) (-47.1062, 38.3182) (-46.8915, 38.2466) (-46.7931, 38.1304) (-46.7931, 38.0588) knots 0 0 0 1 2 3 4 4 4
  line L110 (-46.7931, 38.0588) -> (-46.7931, 29.0973)
  spline S62 degree 2 poles (-28.4416, 31.8752) (-28.4416, 31.1239) (-28.9961, 29.997) (-29.9531, 29.2458) (-31.2231, 28.8612) (-31.9475, 28.8612) knots 0 0 0 1 2 3 4 4 4
  spline S63 degree 2 poles (-31.9475, 28.8612) (-32.4394, 28.8612) (-33.2801, 29.0222) (-33.924, 29.2547) (-34.3623, 29.5051) (-34.5501, 29.6929) (-34.6306, 30.0507) (-34.6306, 30.3906) knots 0 0 0 1 2 3 4 5 6 6 6
  spline S64 degree 2 poles (-34.6306, 30.3906) (-34.6306, 30.6141) (-34.6038, 30.9272) (-34.5322, 31.115) (-34.4249, 31.1955) (-34.3533, 31.1955) knots 0 0 0 1 2 3 4 4 4
  spline S65 degree 2 poles (-34.3533, 31.1955) (-34.246, 31.1955) (-33.8793, 30.954) (-33.289, 30.6589) (-32.4752, 30.4174) (-31.9475, 30.4174) knots 0 0 0 1 2 3 4 4 4
  spline S66 degree 2 poles (-31.9475, 30.4174) (-31.5897, 30.4174) (-31.0352, 30.5873) (-30.6507, 30.8914) (-30.445, 31.3475) (-30.445, 31.6248) knots 0 0 0 1 2 3 4 4 4
  spline S67 degree 2 poles (-30.445, 31.6248) (-30.445, 31.9468) (-30.7938, 32.4118) (-31.3572, 32.7696) (-32.0727, 33.0826) (-32.8419, 33.4314) (-33.5574, 33.8786) (-34.1208, 34.5046) (-34.4696, 35.3543) (-34.4696, 35.9446) knots 0 0 0 1 2 3 4 5 6 7 8 8 8
  spline S68 degree 2 poles (-34.4696, 35.9446) (-34.4696, 36.6332) (-33.9598, 37.6618) (-33.1102, 38.3415) (-31.9386, 38.6813) (-31.2857, 38.6813) knots 0 0 0 1 2 3 4 4 4
  spline S69 degree 2 poles (-31.2857, 38.6813) (-30.9547, 38.6813) (-30.275, 38.5829) (-29.6937, 38.4041) (-29.2376, 38.1805) (-29.0855, 38.0374) (-29.0408, 37.939) (-29.005, 37.7691) (-28.9871, 37.5097) (-28.9871, 37.3219) knots 0 0 0 1 2 3 4 5 6 7 8 8 8
  spline S70 degree 2 poles (-28.9871, 37.3219) (-28.9871, 37.1072) (-29.005, 36.8121) (-29.0587, 36.6243) (-29.1571, 36.5348) (-29.2376, 36.5348) knots 0 0 0 1 2 3 4 4 4
  spline S71 degree 2 poles (-29.2376, 36.5348) (-29.3181, 36.5348) (-29.6669, 36.7406) (-30.1856, 36.982) (-30.8564, 37.1788) (-31.2588, 37.1788) knots 0 0 0 1 2 3 4 4 4
  spline S72 degree 2 poles (-31.2588, 37.1788) (-31.5719, 37.1788) (-32.0459, 37.0268) (-32.3589, 36.7495) (-32.5109, 36.3739) (-32.5109, 36.1592) knots 0 0 0 1 2 3 4 4 4
  spline S73 degree 2 poles (-32.5109, 36.1592) (-32.5109, 35.8462) (-32.1711, 35.3811) (-31.5897, 35.0234) (-30.8564, 34.7103) (-30.0962, 34.3615) (-29.3628, 33.9144) (-28.7904, 33.2883) (-28.4416, 32.4476) (-28.4416, 31.8752) knots 0 0 0 1 2 3 4 5 6 7 8 8 8
  spline S74 degree 2 poles (-9.1537, 37.4963) (-9.1537, 37.2727) (-9.1894, 36.9686) (-9.2699, 36.7987) (-9.3773, 36.7092) (-9.4399, 36.7092) knots 0 0 0 1 2 3 4 4 4
  line L111 (-9.4399, 36.7092) -> (-12.5433, 36.7092)
  line L112 (-12.5433, 36.7092) -> (-12.5433, 34.1603)
  line L113 (-12.5433, 34.1603) -> (-9.6277, 34.1603)
  spline S75 degree 2 poles (-9.6277, 34.1603) (-9.5651, 34.1603) (-9.4577, 34.0887) (-9.3773, 33.9098) (-9.3415, 33.6147) (-9.3415, 33.4001) knots 0 0 0 1 2 3 4 4 4
  spline S76 degree 2 poles (-9.3415, 33.4001) (-9.3415, 33.1765) (-9.3773, 32.8813) (-9.4577, 32.6935) (-9.5651, 32.613) (-9.6277, 32.613) knots 0 0 0 1 2 3 4 4 4
  line L114 (-9.6277, 32.613) -> (-12.5433, 32.613)
  line L115 (-12.5433, 32.613) -> (-12.5433, 29.0803)
  spline S77 degree 2 poles (-12.5433, 29.0803) (-12.5433, 28.9998) (-12.6327, 28.8835) (-12.8563, 28.803) (-13.223, 28.7583) (-13.5092, 28.7583) knots 0 0 0 1 2 3 4 4 4
  spline S78 degree 2 poles (-13.5092, 28.7583) (-13.7865, 28.7583) (-14.1621, 28.803) (-14.3768, 28.8835) (-14.4751, 28.9998) (-14.4751, 29.0803) knots 0 0 0 1 2 3 4 4 4
  line L116 (-14.4751, 29.0803) -> (-14.4751, 37.6751)
  spline S79 degree 2 poles (-14.4751, 37.6751) (-14.4751, 37.9971) (-14.1442, 38.2833) (-13.9027, 38.2833) knots 0 0 0 1 2 2 2
  line L117 (-13.9027, 38.2833) -> (-9.4399, 38.2833)
  spline S80 degree 2 poles (-9.4399, 38.2833) (-9.3773, 38.2833) (-9.2699, 38.2028) (-9.1894, 38.0239) (-9.1537, 37.7109) (-9.1537, 37.4963) knots 0 0 0 1 2 3 4 4 4
  spline S81 degree 2 poles (16.4522, 28.9586) (16.4522, 28.887) (16.3538, 28.7708) (16.1391, 28.6992) (15.7725, 28.6545) (15.4952, 28.6545) knots 0 0 0 1 2 3 4 4 4
  spline S82 degree 2 poles (15.4952, 28.6545) (15.209, 28.6545) (14.8334, 28.6992) (14.6277, 28.7708) (14.5293, 28.887) (14.5293, 28.9586) knots 0 0 0 1 2 3 4 4 4
  line L118 (14.5293, 28.9586) -> (14.5293, 32.7954)
  line L119 (14.5293, 32.7954) -> (10.9697, 32.7954)
  line L120 (10.9697, 32.7954) -> (10.9697, 28.9586)
  spline S83 degree 2 poles (10.9697, 28.9586) (10.9697, 28.887) (10.8803, 28.7708) (10.6656, 28.6992) (10.2989, 28.6545) (10.0127, 28.6545) knots 0 0 0 1 2 3 4 4 4
  spline S84 degree 2 poles (10.0127, 28.6545) (9.7355, 28.6545) (9.3598, 28.6992) (9.1452, 28.7708) (9.0468, 28.887) (9.0468, 28.9586) knots 0 0 0 1 2 3 4 4 4
  line L121 (9.0468, 28.9586) -> (9.0468, 37.9201)
  spline S85 degree 2 poles (9.0468, 37.9201) (9.0468, 37.9917) (9.1452, 38.1079) (9.3598, 38.1795) (9.7355, 38.2242) (10.0127, 38.2242) knots 0 0 0 1 2 3 4 4 4
  spline S86 degree 2 poles (10.0127, 38.2242) (10.2989, 38.2242) (10.6656, 38.1795) (10.8803, 38.1079) (10.9697, 37.9917) (10.9697, 37.9201) knots 0 0 0 1 2 3 4 4 4
  line L122 (10.9697, 37.9201) -> (10.9697, 34.441)
  line L123 (10.9697, 34.441) -> (14.5293, 34.441)
  line L124 (14.5293, 34.441) -> (14.5293, 37.9201)
  spline S87 degree 2 poles (14.5293, 37.9201) (14.5293, 37.9917) (14.6277, 38.1079) (14.8334, 38.1795) (15.209, 38.2242) (15.4952, 38.2242) knots 0 0 0 1 2 3 4 4 4
  spline S88 degree 2 poles (15.4952, 38.2242) (15.7725, 38.2242) (16.1391, 38.1795) (16.3538, 38.1079) (16.4522, 37.9917) (16.4522, 37.9201) knots 0 0 0 1 2 3 4 4 4
  line L125 (16.4522, 37.9201) -> (16.4522, 28.9586)
  spline S89 degree 2 poles (34.8037, 31.7365) (34.8037, 30.9852) (34.2492, 29.8583) (33.2923, 29.1071) (32.0223, 28.7225) (31.2978, 28.7225) knots 0 0 0 1 2 3 4 4 4
  spline S90 degree 2 poles (31.2978, 28.7225) (30.8059, 28.7225) (29.9652, 28.8835) (29.3213, 29.116) (28.883, 29.3664) (28.6952, 29.5542) (28.6147, 29.912) (28.6147, 30.2519) knots 0 0 0 1 2 3 4 5 6 6 6
  spline S91 degree 2 poles (28.6147, 30.2519) (28.6147, 30.4754) (28.6416, 30.7885) (28.7131, 30.9763) (28.8204, 31.0568) (28.892, 31.0568) knots 0 0 0 1 2 3 4 4 4
  spline S92 degree 2 poles (28.892, 31.0568) (28.9993, 31.0568) (29.366, 30.8153) (29.9563, 30.5202) (30.7701, 30.2787) (31.2978, 30.2787) knots 0 0 0 1 2 3 4 4 4
  spline S93 degree 2 poles (31.2978, 30.2787) (31.6556, 30.2787) (32.2101, 30.4486) (32.5947, 30.7527) (32.8004, 31.2088) (32.8004, 31.4861) knots 0 0 0 1 2 3 4 4 4
  spline S94 degree 2 poles (32.8004, 31.4861) (32.8004, 31.808) (32.4516, 32.2731) (31.8881, 32.6309) (31.1726, 32.9439) (30.4035, 33.2927) (29.688, 33.7399) (29.1245, 34.3659) (28.7757, 35.2156) (28.7757, 35.8059) knots 0 0 0 1 2 3 4 5 6 7 8 8 8
  spline S95 degree 2 poles (28.7757, 35.8059) (28.7757, 36.4945) (29.2855, 37.523) (30.1351, 38.2028) (31.3068, 38.5426) (31.9597, 38.5426) knots 0 0 0 1 2 3 4 4 4
  spline S96 degree 2 poles (31.9597, 38.5426) (32.2906, 38.5426) (32.9703, 38.4442) (33.5516, 38.2654) (34.0078, 38.0418) (34.1598, 37.8987) (34.2045, 37.8003) (34.2403, 37.6304) (34.2582, 37.371) (34.2582, 37.1832) knots 0 0 0 1 2 3 4 5 6 7 8 8 8
  spline S97 degree 2 poles (34.2582, 37.1832) (34.2582, 36.9685) (34.2403, 36.6734) (34.1866, 36.4856) (34.0882, 36.3961) (34.0078, 36.3961) knots 0 0 0 1 2 3 4 4 4
  spline S98 degree 2 poles (34.0078, 36.3961) (33.9273, 36.3961) (33.5785, 36.6019) (33.0597, 36.8433) (32.3889, 37.0401) (31.9865, 37.0401) knots 0 0 0 1 2 3 4 4 4
  spline S99 degree 2 poles (31.9865, 37.0401) (31.6735, 37.0401) (31.1994, 36.888) (30.8864, 36.6108) (30.7344, 36.2352) (30.7344, 36.0205) knots 0 0 0 1 2 3 4 4 4
  spline S100 degree 2 poles (30.7344, 36.0205) (30.7344, 35.7075) (31.0742, 35.2424) (31.6556, 34.8847) (32.3889, 34.5716) (33.1492, 34.2228) (33.8825, 33.7757) (34.4549, 33.1496) (34.8037, 32.3089) (34.8037, 31.7365) knots 0 0 0 1 2 3 4 5 6 7 8 8 8
  spline S101 degree 2 poles (54.0917, 37.3576) (54.0917, 37.134) (54.0559, 36.8299) (53.9754, 36.6599) (53.8681, 36.5705) (53.8055, 36.5705) knots 0 0 0 1 2 3 4 4 4
  line L126 (53.8055, 36.5705) -> (50.702, 36.5705)
  line L127 (50.702, 36.5705) -> (50.702, 34.0216)
  line L128 (50.702, 34.0216) -> (53.6176, 34.0216)